Autodesk Inventor part; units mm, degrees
(part 2 of 2)
sketch "Эскиз6" plane through (0, 0, 0) normal (0, 0, -1) x (-1, 0, 0)
  line L0 (-53, 15.6179) -> (-25.3405, 4.0009) projected
  line L1 (-25.3405, 4.0009) -> (-8.0842, -5.3702) projected
  line L2 (-7.9523, -5.3473) -> (-8.0842, -5.3702) projected
  line L3 (-7.789, -5.3433) -> (-7.9523, -5.3473) projected
  line L4 (-7.444, -5.4468) -> (-7.789, -5.3433) projected
  line L5 (-6.7921, -5.8052) -> (-7.444, -5.4468) projected
  line L6 (-6.1197, -6.1235) -> (-6.7921, -5.8052) projected
  line L7 (-5.8336, -6.3424) -> (-6.1197, -6.1235) projected
  line L8 (-5.7412, -6.4771) -> (-5.8336, -6.3424) projected
  line L9 (-5.6824, -6.5974) -> (-5.7412, -6.4771) projected
  line L10 (-5.6419, -6.7101) -> (-5.6824, -6.5974) projected
  line L11 (-5.6135, -6.8178) -> (-5.6419, -6.7101) projected
  line L12 (-5.5818, -7.0232) -> (-5.6135, -6.8178) projected
  line L13 (-5.5741, -7.2193) -> (-5.5818, -7.0232) projected
  line L14 (-5.5841, -7.4089) -> (-5.5741, -7.2193) projected
  line L15 (-5.6083, -7.5933) -> (-5.5841, -7.4089) projected
  line L16 (-5.691, -7.9502) -> (-5.6083, -7.5933) projected
  line L17 (-5.802, -8.2972) -> (-5.691, -7.9502) projected
  line L18 (-5.8532, -8.6645) -> (-5.802, -8.2972) projected
  line L19 (-5.864, -9.0449) -> (-5.8532, -8.6645) projected
  line L20 (-5.8437, -9.4343) -> (-5.864, -9.0449) projected
  line L21 (-5.7962, -9.8308) -> (-5.8437, -9.4343) projected
  line L22 (-5.7233, -10.2331) -> (-5.7962, -9.8308) projected
  line L23 (-5.6263, -10.6399) -> (-5.7233, -10.2331) projected
  line L24 (-5.5062, -11.0504) -> (-5.6263, -10.6399) projected
  line L25 (-5.3633, -11.4634) -> (-5.5062, -11.0504) projected
  line L26 (-5.1983, -11.8783) -> (-5.3633, -11.4634) projected
  line L27 (-5.0602, -12.1901) -> (-5.1983, -11.8783) projected
  line L28 (-2.9375, -12.5288) -> (-5.0602, -12.1901) projected
  line L29 (-2.7092, -12.2754) -> (-2.9375, -12.5288) projected
  line L30 (-2.4233, -11.9325) -> (-2.7092, -12.2754) projected
  line L31 (-2.159, -11.5843) -> (-2.4233, -11.9325) projected
  line L32 (-1.9171, -11.2317) -> (-2.159, -11.5843) projected
  line L33 (-1.6983, -10.8752) -> (-1.9171, -11.2317) projected
  line L34 (-1.5039, -10.5156) -> (-1.6983, -10.8752) projected
  line L35 (-1.3353, -10.1535) -> (-1.5039, -10.5156) projected
  line L36 (-1.1949, -9.7897) -> (-1.3353, -10.1535) projected
  line L37 (-1.0869, -9.4249) -> (-1.1949, -9.7897) projected
  line L38 (-1.0212, -9.0599) -> (-1.0869, -9.4249) projected
  line L39 (-1.0187, -8.6955) -> (-1.0212, -9.0599) projected
  line L40 (-0.9863, -8.3307) -> (-1.0187, -8.6955) projected
  line L41 (-0.9519, -8.1479) -> (-0.9863, -8.3307) projected
  line L42 (-0.9024, -7.9646) -> (-0.9519, -8.1479) projected
  line L43 (-0.834, -7.7806) -> (-0.9024, -7.9646) projected
  line L44 (-0.74, -7.5953) -> (-0.834, -7.7806) projected
  line L45 (-0.6795, -7.5017) -> (-0.74, -7.5953) projected
  line L46 (-0.6059, -7.4072) -> (-0.6795, -7.5017) projected
  line L47 (-0.5127, -7.3112) -> (-0.6059, -7.4072) projected
  line L48 (-0.3829, -7.2119) -> (-0.5127, -7.3112) projected
  line L49 (-0.0429, -7.0929) -> (-0.3829, -7.2119) projected
  line L50 (0.6951, -6.9997) -> (-0.0429, -7.0929) projected
  line L51 (1.4262, -6.8619) -> (0.6951, -6.9997) projected
  line L52 (1.7863, -6.8709) -> (1.4262, -6.8619) projected
  line L53 (1.9402, -6.9255) -> (1.7863, -6.8709) projected
  line L54 (2.0585, -6.9883) -> (1.9402, -6.9255) projected
  line L55 (2.1575, -7.0556) -> (2.0585, -6.9883) projected
  line L56 (2.2438, -7.1261) -> (2.1575, -7.0556) projected
  line L57 (2.3901, -7.2737) -> (2.2438, -7.1261) projected
  line L58 (2.5117, -7.4278) -> (2.3901, -7.2737) projected
  line L59 (2.615, -7.5871) -> (2.5117, -7.4278) projected
  line L60 (2.7039, -7.7505) -> (2.615, -7.5871) projected
  line L61 (2.8467, -8.0877) -> (2.7039, -7.7505) projected
  line L62 (2.9609, -8.4338) -> (2.8467, -8.0877) projected
  line L63 (3.1354, -8.7611) -> (2.9609, -8.4338) projected
  line L64 (3.3502, -9.0751) -> (3.1354, -8.7611) projected
  line L65 (3.5955, -9.3782) -> (3.3502, -9.0751) projected
  line L66 (3.867, -9.6711) -> (3.5955, -9.3782) projected
  line L67 (4.1624, -9.9537) -> (3.867, -9.6711) projected
  line L68 (4.48, -10.2258) -> (4.1624, -9.9537) projected
  line L69 (4.8185, -10.4872) -> (4.48, -10.2258) projected
  line L70 (5.1768, -10.7375) -> (4.8185, -10.4872) projected
  line L71 (5.5542, -10.9761) -> (5.1768, -10.7375) projected
  line L72 (5.8492, -11.1472) -> (5.5542, -10.9761) projected
  line L73 (7.7656, -10.1735) -> (5.8492, -11.1472) projected
  line L74 (7.8013, -9.8343) -> (7.7656, -10.1735) projected
  line L75 (7.8311, -9.3888) -> (7.8013, -9.8343) projected
  line L76 (7.8403, -8.9518) -> (7.8311, -9.3888) projected
  line L77 (7.8287, -8.5243) -> (7.8403, -8.9518) projected
  line L78 (7.7961, -8.1074) -> (7.8287, -8.5243) projected
  line L79 (7.742, -7.7022) -> (7.7961, -8.1074) projected
  line L80 (7.6656, -7.3102) -> (7.742, -7.7022) projected
  line L81 (7.5654, -6.9333) -> (7.6656, -7.3102) projected
  line L82 (7.4384, -6.5746) -> (7.5654, -6.9333) projected
  line L83 (7.2769, -6.2407) -> (7.4384, -6.5746) projected
  line L84 (7.0647, -5.9445) -> (7.2769, -6.2407) projected
  line L85 (6.8765, -5.6303) -> (7.0647, -5.9445) projected
  line L86 (6.7969, -5.4622) -> (6.8765, -5.6303) projected
  line L87 (6.7292, -5.2848) -> (6.7969, -5.4622) projected
  line L88 (6.6764, -5.0958) -> (6.7292, -5.2848) projected
  line L89 (6.6435, -4.8906) -> (6.6764, -5.0958) projected
  line L90 (6.6374, -4.7793) -> (6.6435, -4.8906) projected
  line L91 (6.6415, -4.6596) -> (6.6374, -4.7793) projected
  line L92 (6.6604, -4.5271) -> (6.6415, -4.6596) projected
  line L93 (6.7071, -4.3705) -> (6.6604, -4.5271) projected
  line L94 (6.9122, -4.0744) -> (6.7071, -4.3705) projected
  line L95 (7.4545, -3.5652) -> (6.9122, -4.0744) projected
  line L96 (7.9649, -3.024) -> (7.4545, -3.5652) projected
  line L97 (8.2615, -2.8196) -> (7.9649, -3.024) projected
  line L98 (8.4182, -2.7733) -> (8.2615, -2.8196) projected
  line L99 (8.5508, -2.7546) -> (8.4182, -2.7733) projected
  line L100 (8.6705, -2.7509) -> (8.5508, -2.7546) projected
  line L101 (8.7817, -2.7571) -> (8.6705, -2.7509) projected
  line L102 (8.9868, -2.7905) -> (8.7817, -2.7571) projected
  line L103 (9.1758, -2.8438) -> (8.9868, -2.7905) projected
  line L104 (9.353, -2.9118) -> (9.1758, -2.8438) projected
  line L105 (9.5209, -2.9918) -> (9.353, -2.9118) projected
  line L106 (9.8347, -3.1808) -> (9.5209, -2.9918) projected
  line L107 (10.1304, -3.3936) -> (9.8347, -3.1808) projected
  line L108 (10.464, -3.5558) -> (10.1304, -3.3936) projected
  line L109 (10.8224, -3.6836) -> (10.464, -3.5558) projected
  line L110 (11.199, -3.7847) -> (10.8224, -3.6836) projected
  line L111 (11.5908, -3.862) -> (11.199, -3.7847) projected
  line L112 (11.9959, -3.917) -> (11.5908, -3.862) projected
  line L113 (12.4128, -3.9505) -> (11.9959, -3.917) projected
  line L114 (12.8403, -3.963) -> (12.4128, -3.9505) projected
  line L115 (13.2773, -3.9548) -> (12.8403, -3.963) projected
  line L116 (13.7228, -3.9261) -> (13.2773, -3.9548) projected
  line L117 (14.0621, -3.891) -> (13.7228, -3.9261) projected
  line L118 (15.0401, -1.9769) -> (14.0621, -3.891) projected
  line L119 (14.8697, -1.6815) -> (15.0401, -1.9769) projected
  line L120 (14.6319, -1.3036) -> (14.8697, -1.6815) projected
  line L121 (14.3824, -0.9447) -> (14.6319, -1.3036) projected
  line L122 (14.1218, -0.6056) -> (14.3824, -0.9447) projected
  line L123 (13.8504, -0.2874) -> (14.1218, -0.6056) projected
  line L124 (13.5684, 0.0086) -> (13.8504, -0.2874) projected
  line L125 (13.2762, 0.2808) -> (13.5684, 0.0086) projected
  line L126 (12.9736, 0.5268) -> (13.2762, 0.2808) projected
  line L127 (12.66, 0.7423) -> (12.9736, 0.5268) projected
  line L128 (12.3332, 0.9175) -> (12.66, 0.7423) projected
  line L129 (11.9874, 1.0325) -> (12.3332, 0.9175) projected
  line L130 (11.6504, 1.1761) -> (11.9874, 1.0325) projected
  line L131 (11.4872, 1.2653) -> (11.6504, 1.1761) projected
  line L132 (11.3282, 1.369) -> (11.4872, 1.2653) projected
  line L133 (11.1743, 1.4909) -> (11.3282, 1.369) projected
  line L134 (11.0271, 1.6375) -> (11.1743, 1.4909) projected
  line L135 (10.9568, 1.724) -> (11.0271, 1.6375) projected
  line L136 (10.8897, 1.8232) -> (10.9568, 1.724) projected
  line L137 (10.8272, 1.9416) -> (10.8897, 1.8232) projected
  line L138 (10.7729, 2.0956) -> (10.8272, 1.9416) projected
  line L139 (10.7647, 2.4558) -> (10.7729, 2.0956) projected
  line L140 (10.9042, 3.1865) -> (10.7647, 2.4558) projected
  line L141 (10.999, 3.9243) -> (10.9042, 3.1865) projected
  line L142 (11.1188, 4.264) -> (10.999, 3.9243) projected
  line L143 (11.2183, 4.3936) -> (11.1188, 4.264) projected
  line L144 (11.3146, 4.4866) -> (11.2183, 4.3936) projected
  line L145 (11.4093, 4.56) -> (11.3146, 4.4866) projected
  line L146 (11.5029, 4.6203) -> (11.4093, 4.56) projected
  line L147 (11.6885, 4.7139) -> (11.5029, 4.6203) projected
  line L148 (11.8727, 4.7818) -> (11.6885, 4.7139) projected
  line L149 (12.056, 4.8309) -> (11.8727, 4.7818) projected
  line L150 (12.2389, 4.8649) -> (12.056, 4.8309) projected
  line L151 (12.6038, 4.8965) -> (12.2389, 4.8649) projected
  line L152 (12.9682, 4.8982) -> (12.6038, 4.8965) projected
  line L153 (13.3334, 4.963) -> (12.9682, 4.8982) projected
  line L154 (13.6984, 5.0703) -> (13.3334, 4.963) projected
  line L155 (14.0625, 5.2099) -> (13.6984, 5.0703) projected
  line L156 (14.425, 5.3776) -> (14.0625, 5.2099) projected
  line L157 (14.785, 5.5713) -> (14.425, 5.3776) projected
  line L158 (15.142, 5.7892) -> (14.785, 5.5713) projected
  line L159 (15.4952, 6.0303) -> (15.142, 5.7892) projected
  line L160 (15.8439, 6.2938) -> (15.4952, 6.0303) projected
  line L161 (16.1875, 6.579) -> (15.8439, 6.2938) projected
  line L162 (16.4414, 6.8067) -> (16.1875, 6.579) projected
  line L163 (16.1075, 8.9301) -> (16.4414, 6.8067) projected
  line L164 (15.796, 9.069) -> (16.1075, 8.9301) projected
  line L165 (15.3815, 9.2349) -> (15.796, 9.069) projected
  line L166 (14.9687, 9.3787) -> (15.3815, 9.2349) projected
  line L167 (14.5586, 9.4998) -> (14.9687, 9.3787) projected
  line L168 (14.1519, 9.5976) -> (14.5586, 9.4998) projected
  line L169 (13.7498, 9.6714) -> (14.1519, 9.5976) projected
  line L170 (13.3534, 9.7199) -> (13.7498, 9.6714) projected
  line L171 (12.964, 9.741) -> (13.3534, 9.7199) projected
  line L172 (12.5837, 9.731) -> (12.964, 9.741) projected
  line L173 (12.2162, 9.6807) -> (12.5837, 9.731) projected
  line L174 (11.8689, 9.5704) -> (12.2162, 9.6807) projected
  line L175 (11.5119, 9.4885) -> (11.8689, 9.5704) projected
  line L176 (11.3274, 9.4648) -> (11.5119, 9.4885) projected
  line L177 (11.1379, 9.4552) -> (11.3274, 9.4648) projected
  line L178 (10.9417, 9.4634) -> (11.1379, 9.4552) projected
  line L179 (10.7364, 9.4955) -> (10.9417, 9.4634) projected
  line L180 (10.6287, 9.5241) -> (10.7364, 9.4955) projected
  line L181 (10.5161, 9.5649) -> (10.6287, 9.5241) projected
  line L182 (10.3959, 9.6239) -> (10.5161, 9.5649) projected
  line L183 (10.2615, 9.7167) -> (10.3959, 9.6239) projected
  line L184 (10.0432, 10.0032) -> (10.2615, 9.7167) projected
  line L185 (9.7265, 10.6764) -> (10.0432, 10.0032) projected
  line L186 (9.3696, 11.329) -> (9.7265, 10.6764) projected
  line L187 (9.2668, 11.6743) -> (9.3696, 11.329) projected
  line L188 (9.2712, 11.8376) -> (9.2668, 11.6743) projected
  line L189 (9.2943, 11.9695) -> (9.2712, 11.8376) projected
  line L190 (9.3278, 12.0845) -> (9.2943, 11.9695) projected
  line L191 (9.3681, 12.1883) -> (9.3278, 12.0845) projected
  line L192 (9.4633, 12.3731) -> (9.3681, 12.1883) projected
  line L193 (9.5723, 12.5363) -> (9.4633, 12.3731) projected
  line L194 (9.6918, 12.6838) -> (9.5723, 12.5363) projected
  line L195 (9.8198, 12.8188) -> (9.6918, 12.6838) projected
  line L196 (10.0964, 13.0589) -> (9.8198, 12.8188) projected
  line L197 (10.3902, 13.2744) -> (10.0964, 13.0589) projected
  line L198 (10.6476, 13.5415) -> (10.3902, 13.2744) projected
  line L199 (10.8798, 13.8428) -> (10.6476, 13.5415) projected
  line L200 (11.0924, 14.1698) -> (10.8798, 13.8428) projected
  line L201 (11.1891, 14.3431) -> (11.0924, 14.1698) projected
  arc A0 (11.1891, 14.3431) -> (-16.1963, 14.3431) centre (-2.5036, -3.8906) ccw projected
  arc A1 (-25.3405, 9.161) -> (-16.1963, 14.3431) centre (-40.8164, 47.1281) ccw projected
  line L202 (-25.3405, 9.161) -> (-53, 20.778) projected
  line L203 (-53, 20.778) -> (-57, 20.778) projected
  line L204 (-57, 20.778) -> (-57, 17.5182) projected
  line L205 (-57, 17.5182) -> (-76.2555, 1.8259) projected
  line L206 (-76.2555, 1.8259) -> (-73.7286, -1.2748) projected
  line L207 (-73.7286, -1.2748) -> (-57, 12.3581) projected
  line L208 (-57, 12.3581) -> (-57, -9) projected
  line L209 (-57, -9) -> (-53, -9) projected
  line L210 (-53, -9) -> (-53, 15.6179) projected
  circle A2 centre (-8.3767, 1.5633) radius 1.6 projected
  circle A3 centre (2.3455, -2.0471) radius 1.6 projected
  circle A4 centre (5.9559, 8.675) radius 1.6 projected
  circle A5 centre (-4.7663, 12.2855) radius 1.6 projected
  circle A6 centre (-1.2104, 5.1192) radius 2.5 projected
  line L211 (-57, 17.5182) -> (-57, 12.3581)
  point P0 (0, 0)
  constraints: 2 end point, 1 collinear
extrude "Выдавливание6" cut sketch "Эскиз6" against normal blind 10 contours L207 L206 L205 L211
sketch "Эскиз7" plane through (0, 0, 5) normal (0, 0, 1) x (1, 0, 0)
  line L0 (39.5581, 1.9289) -> (53.904, -11.9897) projected
  line L1 (39.5581, 1.9289) -> (53.904, -11.9897) construction
  line L2 (71.9316, -0.8693) -> (40.2367, -32.4918) construction
  line L3 (71.9316, -0.8693) -> (71.9317, -0.7909) construction
  line L4 (71.9317, -0.7909) -> (40.1893, -0.7429) construction
  line L5 (40.1893, -0.7429) -> (40.1583, -32.5308) construction
  ellipse E0 centre (40.323, 96.1032) end of major axis (40.1583, -32.5308) minor radius 3.174 (40.1583, -32.5308) -> (40.2367, -32.4918) ccw construction
  line L6 (71.9495, -32.6204) -> (72.0099, -0.8302) construction
  ellipse E1 centre (71.7261, -129.4732) end of major axis (71.4423, -258.1162) minor radius 3.1711 (72.0099, -0.8302) -> (71.9316, -0.8693) ccw construction
  line L7 (71.9316, -0.8693) -> (40.2367, -32.4918) construction
  line L8 (40.2367, -32.4918) -> (40.2366, -32.5701) construction
  line L9 (40.2366, -32.5701) -> (71.9495, -32.6204) construction
  line L10 (56.7937, -53.7938) -> (56.9573, -24.3672) projected
  line L11 (56.9573, -24.3672) -> (50.4439, -24.331) projected
  line L12 (50.4439, -24.331) -> (39.4917, -35.2582) projected
  line L13 (39.4917, -35.2582) -> (34.7917, -40.3449) projected
  line L14 (34.7917, -40.3449) -> (19.5374, -31.62) projected
  line L15 (5.5173, -12.5642) -> (19.5374, -31.62) projected
  line L16 (5.5173, -12.5642) -> (5.249, -12.4376) projected
  line L17 (5.0468, -12.5605) -> (5.249, -12.4376) projected
  line L18 (4.7385, -12.7836) -> (5.0468, -12.5605) projected
  line L19 (4.4637, -13.0327) -> (4.7385, -12.7836) projected
  line L20 (4.2394, -13.3198) -> (4.4637, -13.0327) projected
  line L21 (3.9911, -13.589) -> (4.2394, -13.3198) projected
  line L22 (3.8523, -13.7128) -> (3.9911, -13.589) projected
  line L23 (3.7012, -13.8278) -> (3.8523, -13.7128) projected
  line L24 (3.5348, -13.9319) -> (3.7012, -13.8278) projected
  line L25 (3.3472, -14.0213) -> (3.5348, -13.9319) projected
  line L26 (3.2422, -14.0585) -> (3.3472, -14.0213) projected
  line L27 (3.1262, -14.0885) -> (3.2422, -14.0585) projected
  line L28 (2.9937, -14.1076) -> (3.1262, -14.0885) projected
  line L29 (2.8303, -14.1071) -> (2.9937, -14.1076) projected
  line L30 (2.4883, -13.9939) -> (2.8303, -14.1071) projected
  line L31 (1.8468, -13.6173) -> (2.4883, -13.9939) projected
  line L32 (1.1836, -13.2803) -> (1.8468, -13.6173) projected
  line L33 (0.9038, -13.0535) -> (1.1836, -13.2803) projected
  line L34 (0.8152, -12.9162) -> (0.9038, -13.0535) projected
  line L35 (0.7598, -12.7943) -> (0.8152, -12.9162) projected
  line L36 (0.7225, -12.6805) -> (0.7598, -12.7943) projected
  line L37 (0.6971, -12.5721) -> (0.7225, -12.6805) projected
  line L38 (0.6712, -12.3658) -> (0.6971, -12.5721) projected
  line L39 (0.669, -12.1696) -> (0.6712, -12.3658) projected
  line L40 (0.6843, -11.9803) -> (0.669, -12.1696) projected
  line L41 (0.7137, -11.7967) -> (0.6843, -11.9803) projected
  line L42 (0.8064, -11.4423) -> (0.7137, -11.7967) projected
  line L43 (0.9271, -11.0985) -> (0.8064, -11.4423) projected
  line L44 (0.9886, -10.7328) -> (0.9271, -11.0985) projected
  line L45 (1.01, -10.3529) -> (0.9886, -10.7328) projected
  line L46 (1.0007, -9.963) -> (1.01, -10.3529) projected
  line L47 (0.9643, -9.5653) -> (1.0007, -9.963) projected
  line L48 (0.9028, -9.1612) -> (0.9643, -9.5653) projected
  line L49 (0.8173, -8.7518) -> (0.9028, -9.1612) projected
  line L50 (0.7087, -8.3381) -> (0.8173, -8.7518) projected
  line L51 (0.5775, -7.9212) -> (0.7087, -8.3381) projected
  line L52 (0.4242, -7.5019) -> (0.5775, -7.9212) projected
  line L53 (0.2949, -7.1863) -> (0.4242, -7.5019) projected
  line L54 (-1.8175, -6.7882) -> (0.2949, -7.1863) projected
  line L55 (-2.0528, -7.035) -> (-1.8175, -6.7882) projected
  line L56 (-2.3482, -7.3698) -> (-2.0528, -7.035) projected
  line L57 (-2.6222, -7.7104) -> (-2.3482, -7.3698) projected
  line L58 (-2.8739, -8.0561) -> (-2.6222, -7.7104) projected
  line L59 (-3.1025, -8.4063) -> (-2.8739, -8.0561) projected
  line L60 (-3.307, -8.7603) -> (-3.1025, -8.4063) projected
  line L61 (-3.4857, -9.1175) -> (-3.307, -8.7603) projected
  line L62 (-3.6362, -9.4772) -> (-3.4857, -9.1175) projected
  line L63 (-3.7545, -9.8388) -> (-3.6362, -9.4772) projected
  line L64 (-3.8304, -10.2019) -> (-3.7545, -9.8388) projected
  line L65 (-3.8431, -10.566) -> (-3.8304, -10.2019) projected
  line L66 (-3.8858, -10.9298) -> (-3.8431, -10.566) projected
  line L67 (-3.9253, -11.1116) -> (-3.8858, -10.9298) projected
  line L68 (-3.9799, -11.2933) -> (-3.9253, -11.1116) projected
  line L69 (-4.0534, -11.4754) -> (-3.9799, -11.2933) projected
  line L70 (-4.1526, -11.658) -> (-4.0534, -11.4754) projected
  line L71 (-4.2157, -11.7498) -> (-4.1526, -11.658) projected
  line L72 (-4.2919, -11.8422) -> (-4.2157, -11.7498) projected
  line L73 (-4.3879, -11.9356) -> (-4.2919, -11.8422) projected
  line L74 (-4.5203, -12.0312) -> (-4.3879, -11.9356) projected
  line L75 (-4.8636, -12.1406) -> (-4.5203, -12.0312) projected
  line L76 (-5.6039, -12.213) -> (-4.8636, -12.1406) projected
  line L77 (-6.3385, -12.3302) -> (-5.6039, -12.213) projected
  line L78 (-6.6982, -12.3112) -> (-6.3385, -12.3302) projected
  line L79 (-6.8506, -12.2522) -> (-6.6982, -12.3112) projected
  line L80 (-6.967, -12.1861) -> (-6.8506, -12.2522) projected
  line L81 (-7.0642, -12.116) -> (-6.967, -12.1861) projected
  line L82 (-7.1484, -12.0432) -> (-7.0642, -12.116) projected
  line L83 (-7.2906, -11.8916) -> (-7.1484, -12.0432) projected
  line L84 (-7.4077, -11.7341) -> (-7.2906, -11.8916) projected
  line L85 (-7.5066, -11.572) -> (-7.4077, -11.7341) projected
  line L86 (-7.5908, -11.4062) -> (-7.5066, -11.572) projected
  line L87 (-7.7241, -11.065) -> (-7.5908, -11.4062) projected
  line L88 (-7.8285, -10.7159) -> (-7.7241, -11.065) projected
  line L89 (-7.9937, -10.3838) -> (-7.8285, -10.7159) projected
  line L90 (-8.1997, -10.0639) -> (-7.9937, -10.3838) projected
  line L91 (-8.4363, -9.754) -> (-8.1997, -10.0639) projected
  line L92 (-8.6995, -9.4536) -> (-8.4363, -9.754) projected
  line L93 (-8.9869, -9.1628) -> (-8.6995, -9.4536) projected
  line L94 (-9.2967, -8.8819) -> (-8.9869, -9.1628) projected
  line L95 (-9.6277, -8.6111) -> (-9.2967, -8.8819) projected
  line L96 (-9.9789, -8.3509) -> (-9.6277, -8.6111) projected
  line L97 (-10.3494, -8.1017) -> (-9.9789, -8.3509) projected
  line L98 (-10.6395, -7.9224) -> (-10.3494, -8.1017) projected
  line L99 (-12.5824, -8.8419) -> (-10.6395, -7.9224) projected
  line L100 (-12.6277, -9.18) -> (-12.5824, -8.8419) projected
  line L101 (-12.67, -9.6245) -> (-12.6277, -9.18) projected
  line L102 (-12.6914, -10.061) -> (-12.67, -9.6245) projected
  line L103 (-12.6918, -10.4887) -> (-12.6914, -10.061) projected
  line L104 (-12.671, -10.9064) -> (-12.6918, -10.4887) projected
  line L105 (-12.6283, -11.3129) -> (-12.671, -10.9064) projected
  line L106 (-12.5629, -11.7069) -> (-12.6283, -11.3129) projected
  line L107 (-12.4733, -12.0864) -> (-12.5629, -11.7069) projected
  line L108 (-12.3564, -12.4485) -> (-12.4733, -12.0864) projected
  line L109 (-12.2044, -12.7869) -> (-12.3564, -12.4485) projected
  line L110 (-12.0007, -13.0889) -> (-12.2044, -12.7869) projected
  line L111 (-11.8213, -13.4083) -> (-12.0007, -13.0889) projected
  line L112 (-11.7465, -13.5786) -> (-11.8213, -13.4083) projected
  line L113 (-11.6838, -13.7578) -> (-11.7465, -13.5786) projected
  line L114 (-11.6363, -13.9482) -> (-11.6838, -13.7578) projected
  line L115 (-11.6092, -14.1543) -> (-11.6363, -13.9482) projected
  line L116 (-11.6063, -14.2657) -> (-11.6092, -14.1543) projected
  line L117 (-11.6136, -14.3852) -> (-11.6063, -14.2657) projected
  line L118 (-11.6363, -14.5171) -> (-11.6136, -14.3852) projected
  line L119 (-11.6874, -14.6723) -> (-11.6363, -14.5171) projected
  line L120 (-11.9007, -14.9626) -> (-11.6874, -14.6723) projected
  line L121 (-12.4571, -15.4564) -> (-11.9007, -14.9626) projected
  line L122 (-12.9825, -15.983) -> (-12.4571, -15.4564) projected
  line L123 (-13.2847, -16.179) -> (-12.9825, -15.983) projected
  line L124 (-13.4426, -16.2209) -> (-13.2847, -16.179) projected
  line L125 (-13.5757, -16.2359) -> (-13.4426, -16.2209) projected
  line L126 (-13.6954, -16.2362) -> (-13.5757, -16.2359) projected
  line L127 (-13.8065, -16.2268) -> (-13.6954, -16.2362) projected
  line L128 (-14.0106, -16.1877) -> (-13.8065, -16.2268) projected
  line L129 (-14.1979, -16.1291) -> (-14.0106, -16.1877) projected
  line L130 (-14.3731, -16.0561) -> (-14.1979, -16.1291) projected
  line L131 (-14.5388, -15.9714) -> (-14.3731, -16.0561) projected
  line L132 (-14.8471, -15.7738) -> (-14.5388, -15.9714) projected
  line L133 (-15.1368, -15.5527) -> (-14.8471, -15.7738) projected
  line L134 (-15.4657, -15.3812) -> (-15.1368, -15.5527) projected
  line L135 (-15.8203, -15.2434) -> (-15.4657, -15.3812) projected
  line L136 (-16.1939, -15.1318) -> (-15.8203, -15.2434) projected
  line L137 (-16.5834, -15.0435) -> (-16.1939, -15.1318) projected
  line L138 (-16.9868, -14.9772) -> (-16.5834, -15.0435) projected
  line L139 (-17.4026, -14.932) -> (-16.9868, -14.9772) projected
  line L140 (-17.8296, -14.9074) -> (-17.4026, -14.932) projected
  line L141 (-18.2666, -14.9033) -> (-17.8296, -14.9074) projected
  line L142 (-18.7128, -14.9196) -> (-18.2666, -14.9033) projected
  line L143 (-19.0529, -14.945) -> (-18.7128, -14.9196) projected
  line L144 (-20.0843, -16.831) -> (-19.0529, -14.945) projected
  line L145 (-19.9222, -17.1311) -> (-20.0843, -16.831) projected
  line L146 (-19.6952, -17.5155) -> (-19.9222, -17.1311) projected
  line L147 (-19.4559, -17.8813) -> (-19.6952, -17.5155) projected
  line L148 (-19.2049, -18.2275) -> (-19.4559, -17.8813) projected
  line L149 (-18.9425, -18.5532) -> (-19.2049, -18.2275) projected
  line L150 (-18.669, -18.857) -> (-18.9425, -18.5532) projected
  line L151 (-18.3845, -19.1373) -> (-18.669, -18.857) projected
  line L152 (-18.0889, -19.3917) -> (-18.3845, -19.1373) projected
  line L153 (-17.7816, -19.6159) -> (-18.0889, -19.3917) projected
  line L154 (-17.4597, -19.8003) -> (-17.7816, -19.6159) projected
  line L155 (-17.1173, -19.9249) -> (-17.4597, -19.8003) projected
  line L156 (-16.7845, -20.0779) -> (-17.1173, -19.9249) projected
  line L157 (-16.6239, -20.1717) -> (-16.7845, -20.0779) projected
  line L158 (-16.4679, -20.2798) -> (-16.6239, -20.1717) projected
  line L159 (-16.3175, -20.4059) -> (-16.4679, -20.2798) projected
  line L160 (-16.1744, -20.5567) -> (-16.3175, -20.4059) projected
  line L161 (-16.1066, -20.6451) -> (-16.1744, -20.5567) projected
  line L162 (-16.0423, -20.7461) -> (-16.1066, -20.6451) projected
  line L163 (-15.9831, -20.8662) -> (-16.0423, -20.7461) projected
  line L164 (-15.9331, -21.0218) -> (-15.9831, -20.8662) projected
  line L165 (-15.9351, -21.382) -> (-15.9331, -21.0218) projected
  line L166 (-16.095, -22.1085) -> (-15.9351, -21.382) projected
  line L167 (-16.2106, -22.8433) -> (-16.095, -22.1085) projected
  line L168 (-16.3398, -23.1796) -> (-16.2106, -22.8433) projected
  line L169 (-16.443, -23.3063) -> (-16.3398, -23.1796) projected
  line L170 (-16.5418, -23.3966) -> (-16.443, -23.3063) projected
  line L171 (-16.6385, -23.4673) -> (-16.5418, -23.3966) projected
  line L172 (-16.7338, -23.5249) -> (-16.6385, -23.4673) projected
  line L173 (-16.922, -23.6132) -> (-16.7338, -23.5249) projected
  line L174 (-17.108, -23.676) -> (-16.922, -23.6132) projected
  line L175 (-17.2926, -23.7199) -> (-17.108, -23.676) projected
  line L176 (-17.4764, -23.7488) -> (-17.2926, -23.7199) projected
  line L177 (-17.842, -23.7701) -> (-17.4764, -23.7488) projected
  line L178 (-18.2063, -23.7615) -> (-17.842, -23.7701) projected
  line L179 (-18.5732, -23.8161) -> (-18.2063, -23.7615) projected
  line L180 (-18.9411, -23.9131) -> (-18.5732, -23.8161) projected
  line L181 (-19.309, -24.0423) -> (-18.9411, -23.9131) projected
  line L182 (-19.676, -24.1999) -> (-19.309, -24.0423) projected
  line L183 (-20.0413, -24.3833) -> (-19.676, -24.1999) projected
  line L184 (-20.4043, -24.5911) -> (-20.0413, -24.3833) projected
  line L185 (-20.7641, -24.8222) -> (-20.4043, -24.5911) projected
  line L186 (-20.9152, -24.9299) -> (-20.7641, -24.8222) projected
  arc A0 (-20.9152, -24.9299) -> (6.9816, -38.099) centre (0.2024, -16.3274) ccw projected
  arc A1 (17.3347, -36.2863) -> (6.9816, -38.099) centre (19.1709, -77.2451) ccw projected
  line L187 (17.3347, -36.2863) -> (47.4599, -51.9843) projected
  line L188 (47.4599, -51.9843) -> (52.9562, -54.744) projected
  line L189 (52.9562, -54.744) -> (56.7937, -53.7938) projected
  circle A2 centre (-3.0949, -32.3247) radius 1.6 projected
  circle A3 centre (3.9045, -23.436) radius 1.6 projected
  circle A4 centre (-4.9841, -16.4366) radius 1.6 projected
  circle A5 centre (-4.0395, -24.3806) radius 2.5 projected
  circle A6 centre (-11.9836, -25.3252) radius 1.6 projected
  line L190 (40.1738, -16.6369) -> (71.9797, -16.7253)
  ellipse E2 centre (39.6963, -129.376) end of major axis (40.2467, -0.7431) minor radius 3.174 (40.3248, -0.7826) -> (40.2467, -0.7431) ccw construction
  line L191 (40.3248, -0.7826) -> (40.3251, -0.7042) construction
  line L192 (57, 20.4271) -> (57, -9)
  line L193 (57, -9) -> (50.4865, -9)
  line L194 (50.4865, -9) -> (39.5953, 1.9879)
  line L195 (39.5953, 1.9879) -> (34.3127, 7.7692)
  line L196 (47.6562, 18.6694) -> (53.1678, 21.3986)
  line L197 (53.1678, 21.3986) -> (57, 20.4271)
  line L198 (53, 15.6179) -> (25.3405, 4.0009) projected
  circle A7 centre (8.3767, 1.5633) radius 1.6 projected
  circle A8 centre (-2.3455, -2.0471) radius 1.6 projected
  circle A9 centre (-5.9559, 8.675) radius 1.6 projected
  circle A10 centre (4.7663, 12.2855) radius 1.6 projected
  circle A11 centre (1.2104, 5.1192) radius 2.5 projected
  line L199 (57, -9) -> (57, 20.778) projected
  line L200 (53, 20.778) -> (57, 20.778) projected
  line L201 (25.3405, 9.161) -> (53, 20.778) projected
  arc A12 (16.1963, 14.3431) -> (25.3405, 9.161) centre (40.8164, 47.1281) ccw projected
  arc A13 (16.1963, 14.3431) -> (-11.1891, 14.3431) centre (2.5036, -3.8906) ccw projected
  line L202 (-11.1891, 14.3431) -> (-11.0924, 14.1698) projected
  line L203 (-11.0924, 14.1698) -> (-10.8798, 13.8428) projected
  line L204 (-10.8798, 13.8428) -> (-10.6476, 13.5415) projected
  line L205 (-10.6476, 13.5415) -> (-10.3902, 13.2744) projected
  line L206 (-10.3902, 13.2744) -> (-10.0964, 13.0589) projected
  line L207 (-10.0964, 13.0589) -> (-9.8198, 12.8188) projected
  line L208 (-9.8198, 12.8188) -> (-9.6918, 12.6838) projected
  line L209 (-9.6918, 12.6838) -> (-9.5723, 12.5363) projected
  line L210 (-9.5723, 12.5363) -> (-9.4633, 12.3731) projected
  line L211 (-9.4633, 12.3731) -> (-9.3681, 12.1883) projected
  line L212 (-9.3681, 12.1883) -> (-9.3278, 12.0845) projected
  line L213 (-9.3278, 12.0845) -> (-9.2943, 11.9695) projected
  line L214 (-9.2943, 11.9695) -> (-9.2712, 11.8376) projected
  line L215 (-9.2712, 11.8376) -> (-9.2668, 11.6743) projected
  line L216 (-9.2668, 11.6743) -> (-9.3696, 11.329) projected
  line L217 (-9.3696, 11.329) -> (-9.7265, 10.6764) projected
  line L218 (-9.7265, 10.6764) -> (-10.0432, 10.0032) projected
  line L219 (-10.0432, 10.0032) -> (-10.2615, 9.7167) projected
  line L220 (-10.2615, 9.7167) -> (-10.3959, 9.6239) projected
  line L221 (-10.3959, 9.6239) -> (-10.5161, 9.5649) projected
  line L222 (-10.5161, 9.5649) -> (-10.6287, 9.5241) projected
  line L223 (-10.6287, 9.5241) -> (-10.7364, 9.4955) projected
  line L224 (-10.7364, 9.4955) -> (-10.9417, 9.4634) projected
  line L225 (-10.9417, 9.4634) -> (-11.1379, 9.4552) projected
  line L226 (-11.1379, 9.4552) -> (-11.3274, 9.4648) projected
  line L227 (-11.3274, 9.4648) -> (-11.5119, 9.4885) projected
  line L228 (-11.5119, 9.4885) -> (-11.8689, 9.5704) projected
  line L229 (-11.8689, 9.5704) -> (-12.2162, 9.6807) projected
  line L230 (-12.2162, 9.6807) -> (-12.5837, 9.731) projected
  line L231 (-12.5837, 9.731) -> (-12.964, 9.741) projected
  line L232 (-12.964, 9.741) -> (-13.3534, 9.7199) projected
  line L233 (-13.3534, 9.7199) -> (-13.7498, 9.6714) projected
  line L234 (-13.7498, 9.6714) -> (-14.1519, 9.5976) projected
  line L235 (-14.1519, 9.5976) -> (-14.5586, 9.4998) projected
  line L236 (-14.5586, 9.4998) -> (-14.9687, 9.3787) projected
  line L237 (-14.9687, 9.3787) -> (-15.3815, 9.2349) projected
  line L238 (-15.3815, 9.2349) -> (-15.796, 9.069) projected
  line L239 (-15.796, 9.069) -> (-16.1075, 8.9301) projected
  line L240 (-16.1075, 8.9301) -> (-16.4414, 6.8067) projected
  line L241 (-16.4414, 6.8067) -> (-16.1875, 6.579) projected
  line L242 (-16.1875, 6.579) -> (-15.8439, 6.2938) projected
  line L243 (-15.8439, 6.2938) -> (-15.4952, 6.0303) projected
  line L244 (-15.4952, 6.0303) -> (-15.142, 5.7892) projected
  line L245 (-15.142, 5.7892) -> (-14.785, 5.5713) projected
  line L246 (-14.785, 5.5713) -> (-14.425, 5.3776) projected
  line L247 (-14.425, 5.3776) -> (-14.0625, 5.2099) projected
  line L248 (-14.0625, 5.2099) -> (-13.6984, 5.0703) projected
  line L249 (-13.6984, 5.0703) -> (-13.3334, 4.963) projected
  line L250 (-13.3334, 4.963) -> (-12.9682, 4.8982) projected
  line L251 (-12.9682, 4.8982) -> (-12.6038, 4.8965) projected
  line L252 (-12.6038, 4.8965) -> (-12.2389, 4.8649) projected
  line L253 (-12.2389, 4.8649) -> (-12.056, 4.8309) projected
  line L254 (-12.056, 4.8309) -> (-11.8727, 4.7818) projected
  line L255 (-11.8727, 4.7818) -> (-11.6885, 4.7139) projected
  line L256 (-11.6885, 4.7139) -> (-11.5029, 4.6203) projected
  line L257 (-11.5029, 4.6203) -> (-11.4093, 4.56) projected
  line L258 (-11.4093, 4.56) -> (-11.3146, 4.4866) projected
  line L259 (-11.3146, 4.4866) -> (-11.2183, 4.3936) projected
  line L260 (-11.2183, 4.3936) -> (-11.1188, 4.264) projected
  line L261 (-11.1188, 4.264) -> (-10.999, 3.9243) projected
  line L262 (-10.999, 3.9243) -> (-10.9042, 3.1865) projected
  line L263 (-10.9042, 3.1865) -> (-10.7647, 2.4558) projected
  line L264 (-10.7647, 2.4558) -> (-10.7729, 2.0956) projected
  line L265 (-10.7729, 2.0956) -> (-10.8272, 1.9416) projected
  line L266 (-10.8272, 1.9416) -> (-10.8897, 1.8232) projected
  line L267 (-10.8897, 1.8232) -> (-10.9568, 1.724) projected
  line L268 (-10.9568, 1.724) -> (-11.0271, 1.6375) projected
  line L269 (-11.0271, 1.6375) -> (-11.1743, 1.4909) projected
  line L270 (-11.1743, 1.4909) -> (-11.3282, 1.369) projected
  line L271 (-11.3282, 1.369) -> (-11.4872, 1.2653) projected
  line L272 (-11.4872, 1.2653) -> (-11.6504, 1.1761) projected
  line L273 (-11.6504, 1.1761) -> (-11.9874, 1.0325) projected
  line L274 (-11.9874, 1.0325) -> (-12.3332, 0.9175) projected
  line L275 (-12.3332, 0.9175) -> (-12.66, 0.7423) projected
  line L276 (-12.66, 0.7423) -> (-12.9736, 0.5268) projected
  line L277 (-12.9736, 0.5268) -> (-13.2762, 0.2808) projected
  line L278 (-13.2762, 0.2808) -> (-13.5684, 0.0086) projected
  line L279 (-13.5684, 0.0086) -> (-13.8504, -0.2874) projected
  line L280 (-13.8504, -0.2874) -> (-14.1218, -0.6056) projected
  line L281 (-14.1218, -0.6056) -> (-14.3824, -0.9447) projected
  line L282 (-14.3824, -0.9447) -> (-14.6319, -1.3036) projected
  line L283 (-14.6319, -1.3036) -> (-14.8697, -1.6815) projected
  line L284 (-14.8697, -1.6815) -> (-15.0401, -1.9769) projected
  line L285 (-15.0401, -1.9769) -> (-14.0621, -3.891) projected
  line L286 (-14.0621, -3.891) -> (-13.7228, -3.9261) projected
  line L287 (-13.7228, -3.9261) -> (-13.2773, -3.9548) projected
  line L288 (-13.2773, -3.9548) -> (-12.8403, -3.963) projected
  line L289 (-12.8403, -3.963) -> (-12.4128, -3.9505) projected
  line L290 (-12.4128, -3.9505) -> (-11.9959, -3.917) projected
  line L291 (-11.9959, -3.917) -> (-11.5908, -3.862) projected
  line L292 (-11.5908, -3.862) -> (-11.199, -3.7847) projected
  line L293 (-11.199, -3.7847) -> (-10.8224, -3.6836) projected
  line L294 (-10.8224, -3.6836) -> (-10.464, -3.5558) projected
  line L295 (-10.464, -3.5558) -> (-10.1304, -3.3936) projected
  line L296 (-10.1304, -3.3936) -> (-9.8347, -3.1808) projected
  line L297 (-9.8347, -3.1808) -> (-9.5209, -2.9918) projected
  line L298 (-9.5209, -2.9918) -> (-9.353, -2.9118) projected
  line L299 (-9.353, -2.9118) -> (-9.1758, -2.8438) projected
  line L300 (-9.1758, -2.8438) -> (-8.9868, -2.7905) projected
  line L301 (-8.9868, -2.7905) -> (-8.7817, -2.7571) projected
  line L302 (-8.7817, -2.7571) -> (-8.6705, -2.7509) projected
  line L303 (-8.6705, -2.7509) -> (-8.5508, -2.7546) projected
  line L304 (-8.5508, -2.7546) -> (-8.4182, -2.7733) projected
  line L305 (-8.4182, -2.7733) -> (-8.2615, -2.8196) projected
  line L306 (-8.2615, -2.8196) -> (-7.9649, -3.024) projected
  line L307 (-7.9649, -3.024) -> (-7.4545, -3.5652) projected
  line L308 (-7.4545, -3.5652) -> (-6.9122, -4.0744) projected
  line L309 (-6.9122, -4.0744) -> (-6.7071, -4.3705) projected
  line L310 (-6.7071, -4.3705) -> (-6.6604, -4.5271) projected
  line L311 (-6.6604, -4.5271) -> (-6.6415, -4.6596) projected
  line L312 (-6.6415, -4.6596) -> (-6.6374, -4.7793) projected
  line L313 (-6.6374, -4.7793) -> (-6.6435, -4.8906) projected
  line L314 (-6.6435, -4.8906) -> (-6.6764, -5.0958) projected
  line L315 (-6.6764, -5.0958) -> (-6.7292, -5.2848) projected
  line L316 (-6.7292, -5.2848) -> (-6.7969, -5.4622) projected
  line L317 (-6.7969, -5.4622) -> (-6.8765, -5.6303) projected
  line L318 (-6.8765, -5.6303) -> (-7.0647, -5.9445) projected
  line L319 (-7.0647, -5.9445) -> (-7.2769, -6.2407) projected
  line L320 (-7.2769, -6.2407) -> (-7.4384, -6.5746) projected
  line L321 (-7.4384, -6.5746) -> (-7.5654, -6.9333) projected
  line L322 (-7.5654, -6.9333) -> (-7.6656, -7.3102) projected
  line L323 (-7.6656, -7.3102) -> (-7.742, -7.7022) projected
  line L324 (-7.742, -7.7022) -> (-7.7961, -8.1074) projected
  line L325 (-7.7961, -8.1074) -> (-7.8287, -8.5243) projected
  line L326 (-7.8287, -8.5243) -> (-7.8403, -8.9518) projected
  line L327 (-7.8403, -8.9518) -> (-7.8311, -9.3888) projected
  line L328 (-7.8311, -9.3888) -> (-7.8013, -9.8343) projected
  line L329 (-7.8013, -9.8343) -> (-7.7656, -10.1735) projected
  line L330 (-7.7656, -10.1735) -> (-5.8492, -11.1472) projected
  line L331 (-5.8492, -11.1472) -> (-5.5542, -10.9761) projected
  line L332 (-5.5542, -10.9761) -> (-5.1768, -10.7375) projected
  line L333 (-5.1768, -10.7375) -> (-4.8185, -10.4872) projected
  line L334 (-4.8185, -10.4872) -> (-4.48, -10.2258) projected
  line L335 (-4.48, -10.2258) -> (-4.1624, -9.9537) projected
  line L336 (-4.1624, -9.9537) -> (-3.867, -9.6711) projected
  line L337 (-3.867, -9.6711) -> (-3.5955, -9.3782) projected
  line L338 (-3.5955, -9.3782) -> (-3.3502, -9.0751) projected
  line L339 (-3.3502, -9.0751) -> (-3.1354, -8.7611) projected
  line L340 (-3.1354, -8.7611) -> (-2.9609, -8.4338) projected
  line L341 (-2.9609, -8.4338) -> (-2.8467, -8.0877) projected
  line L342 (-2.8467, -8.0877) -> (-2.7039, -7.7505) projected
  line L343 (-2.7039, -7.7505) -> (-2.615, -7.5871) projected
  line L344 (-2.615, -7.5871) -> (-2.5117, -7.4278) projected
  line L345 (-2.5117, -7.4278) -> (-2.3901, -7.2737) projected
  line L346 (-2.3901, -7.2737) -> (-2.2438, -7.1261) projected
  line L347 (-2.2438, -7.1261) -> (-2.1575, -7.0556) projected
  line L348 (-2.1575, -7.0556) -> (-2.0585, -6.9883) projected
  line L349 (-2.0585, -6.9883) -> (-1.9402, -6.9255) projected
  line L350 (-1.9402, -6.9255) -> (-1.7863, -6.8709) projected
  line L351 (-1.7863, -6.8709) -> (-1.4262, -6.8619) projected
  line L352 (-1.4262, -6.8619) -> (-0.6951, -6.9997) projected
  line L353 (-0.6951, -6.9997) -> (0.0429, -7.0929) projected
  line L354 (0.0429, -7.0929) -> (0.3829, -7.2119) projected
  line L355 (0.3829, -7.2119) -> (0.5127, -7.3112) projected
  line L356 (0.5127, -7.3112) -> (0.6059, -7.4072) projected
  line L357 (0.6059, -7.4072) -> (0.6795, -7.5017) projected
  line L358 (0.6795, -7.5017) -> (0.74, -7.5953) projected
  line L359 (0.74, -7.5953) -> (0.834, -7.7806) projected
  line L360 (0.834, -7.7806) -> (0.9024, -7.9646) projected
  line L361 (0.9024, -7.9646) -> (0.9519, -8.1479) projected
  line L362 (0.9519, -8.1479) -> (0.9863, -8.3307) projected
  line L363 (0.9863, -8.3307) -> (1.0187, -8.6955) projected
  line L364 (1.0187, -8.6955) -> (1.0212, -9.0599) projected
  line L365 (1.0212, -9.0599) -> (1.0869, -9.4249) projected
  line L366 (1.0869, -9.4249) -> (1.1949, -9.7897) projected
  line L367 (1.1949, -9.7897) -> (1.3353, -10.1535) projected
  line L368 (1.3353, -10.1535) -> (1.5039, -10.5156) projected
  line L369 (1.5039, -10.5156) -> (1.6983, -10.8752) projected
  line L370 (1.6983, -10.8752) -> (1.9171, -11.2317) projected
  line L371 (1.9171, -11.2317) -> (2.159, -11.5843) projected
  line L372 (2.159, -11.5843) -> (2.4233, -11.9325) projected
  line L373 (2.4233, -11.9325) -> (2.7092, -12.2754) projected
  line L374 (2.7092, -12.2754) -> (2.9375, -12.5288) projected
  line L375 (2.9375, -12.5288) -> (5.0602, -12.1901) projected
  line L376 (5.0602, -12.1901) -> (5.1983, -11.8783) projected
  line L377 (5.1983, -11.8783) -> (5.3633, -11.4634) projected
  line L378 (5.3633, -11.4634) -> (5.5062, -11.0504) projected
  line L379 (5.5062, -11.0504) -> (5.6263, -10.6399) projected
  line L380 (5.6263, -10.6399) -> (5.7233, -10.2331) projected
  line L381 (5.7233, -10.2331) -> (5.7962, -9.8308) projected
  line L382 (5.7962, -9.8308) -> (5.8437, -9.4343) projected
  line L383 (5.8437, -9.4343) -> (5.864, -9.0449) projected
  line L384 (5.864, -9.0449) -> (5.8532, -8.6645) projected
  line L385 (5.8532, -8.6645) -> (5.802, -8.2972) projected
  line L386 (5.802, -8.2972) -> (5.691, -7.9502) projected
  line L387 (5.691, -7.9502) -> (5.6083, -7.5933) projected
  line L388 (5.6083, -7.5933) -> (5.5841, -7.4089) projected
  line L389 (5.5841, -7.4089) -> (5.5741, -7.2193) projected
  line L390 (5.5741, -7.2193) -> (5.5818, -7.0232) projected
  line L391 (5.5818, -7.0232) -> (5.6135, -6.8178) projected
  line L392 (5.6135, -6.8178) -> (5.6419, -6.7101) projected
  line L393 (5.6419, -6.7101) -> (5.6824, -6.5974) projected
  line L394 (5.6824, -6.5974) -> (5.7412, -6.4771) projected
  line L395 (5.7412, -6.4771) -> (5.8336, -6.3424) projected
  line L396 (5.8336, -6.3424) -> (6.1197, -6.1235) projected
  line L397 (6.1197, -6.1235) -> (6.7921, -5.8052) projected
  line L398 (6.7921, -5.8052) -> (7.444, -5.4468) projected
  line L399 (7.444, -5.4468) -> (7.789, -5.3433) projected
  line L400 (7.789, -5.3433) -> (7.9523, -5.3473) projected
  line L401 (7.9523, -5.3473) -> (8.0842, -5.3702) projected
  line L402 (8.0842, -5.3702) -> (25.3405, 4.0009) projected
  line L403 (53, 15.6179) -> (25.3405, 4.0009) projected
  line L404 (53, -9) -> (53, 15.6179) projected
  line L405 (57, -9) -> (53, -9) projected
  point P0 (0, 0)
  point P1 (53.878, -21.3603)
  point P2 (34.9235, 7.1007)
  point P3 (42.0547, -0.4934)
  point P4 (50.8225, -9)
  constraints: 16 end point, 12 symmetric about line, 2 midpoint, 2 point on line, 7 other
extrude "Выдавливание7" add sketch "Эскиз7" against normal up to surface (5 mm away) contours L194 L195 L198 L404 L193 L0
